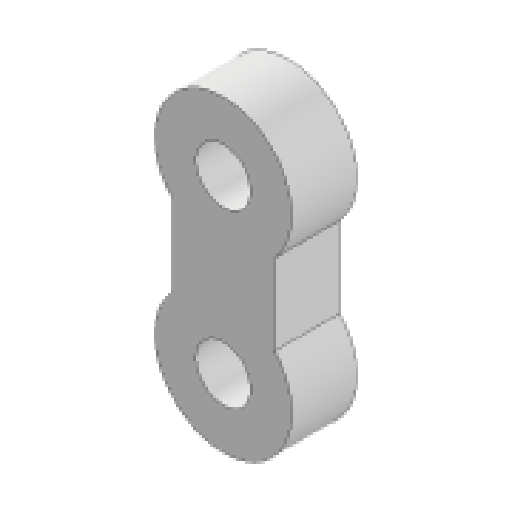
# Autodesk Inventor part: Arm 1
Saved by Autodesk Inventor 2025 (Build 290162010, 162A)
## iProperties
Created: 2024-11-29
Part Number: Arm 1
Material: Generic
Document SubType Name: Modeling
Designer: alexa
Density: 1 g/cm^3
Appearance: Default
Author: alexa
Autodesk Inventor part; units mm, degrees
ref_plane "YZ Plane" through (0, 0, 0) normal (1, 0, 0) x (0, 1, 0)
ref_plane "XZ Plane" through (0, 0, 0) normal (0, 1, 0) x (-1, 0, 0)
ref_plane "XY Plane" through (0, 0, 0) normal (0, 0, 1) x (1, 0, 0)
sketch "Sketch1" plane through (0, 0, 0) normal (0, 0, 1) x (1, 0, 0)
  circle A0 centre (0, 0) radius 2.032
  arc A1 (-3.81, 3.3601) -> (3.81, 3.3601) centre (0, 0) ccw
  line L0 (-3.81, 3.3601) -> (-3.81, 9.3399)
  circle A2 centre (0, 12.7) radius 2.032
  arc A3 (3.81, 9.3399) -> (-3.81, 9.3399) centre (0, 12.7) ccw
  line L1 (3.81, 9.3399) -> (3.81, 3.3601)
  point P0 (-3.81, 6.35)
  dimension "d0" = 4.064
  dimension "d1" = 10.16
  dimension "d3" = 4.064
  dimension "d5" = 12.7
  dimension "d31" = 5.08
  dimension "d34" = 7.62
  dimension "d35" = 3.81
  constraints: 4 centre point, 4 end point, 4 point on circle, 3 coincident, 2 vertical, 1 midpoint, 1 vertical alignment
  measures "d0" diameter of A0
  measures "d1" diameter of A1
  measures "d3" diameter of A2
  measures "d5" distance of point (0, 0) A2.centre
  measures "d31" radius of A3
  measures "d34" distance between parallel lines of L0 L1
  measures "d35" distance from line of point (0, 0) L0
extrude "Extrusion1" add sketch "Sketch1" along normal blind 4.826
equation "\"d0\" = d3"
equation "\"d35\" = 0.5 * d34"
body "Solid1"
